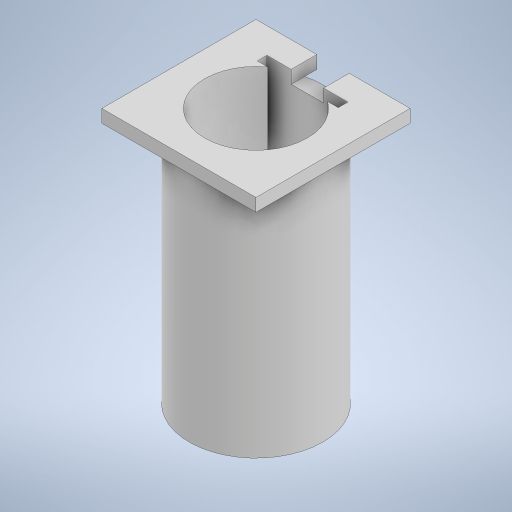
# Autodesk Inventor part: WaterBucket2
Saved by Autodesk Inventor 2023 (Build 270158000, 158)
## iProperties
Created: 2023-11-16
Part Number: WaterBucket2
Material: Generic
Document SubType Name: Modeling
Designer: Gage
Density: 1 g/cm^3
Appearance: Default
Author: Gage
Autodesk Inventor part; units mm, degrees
ref_plane "YZ Plane" through (0, 0, 0) normal (1, 0, 0) x (0, 1, 0)
ref_plane "XZ Plane" through (0, 0, 0) normal (0, 1, 0) x (-1, 0, 0)
ref_plane "XY Plane" through (0, 0, 0) normal (0, 0, 1) x (1, 0, 0)
sketch "Sketch1" plane through (0, 0, 0) normal (0, 1, 0) x (-1, 0, 0)
  circle A0 centre (0, 0) radius 16.51
  dimension "d0" = 33.02
  constraints: 1 centre point, 1 coincident
  measures "d0" diameter of A0
extrude "Extrusion1" add sketch "Sketch1" along normal blind 58.42
sketch "Sketch3" plane through (0, 58.42, 0) normal (0, 1, 0) x (1, 0, 0)
  line L0 (-19.05, 19.05) -> (19.05, 19.05)
  line L1 (19.05, 19.05) -> (19.05, -19.05)
  line L2 (19.05, -19.05) -> (-19.05, -19.05)
  line L3 (-19.05, -19.05) -> (-19.05, 19.05)
  point P0 (0, 0)
  point P1 (19.05, 0)
  point P2 (0, 19.05)
  dimension "d8" = 38.1
  dimension "d9" = 38.1
  constraints: 8 end point, 2 midpoint, 2 parallel, 1 horizontal, 1 horizontal alignment, 1 perpendicular, 1 vertical alignment
  measures "d8" distance of L1.end L2.end
  measures "d9" distance of L0.end L1.end
extrude "Extrusion3" add sketch "Sketch3" along normal blind 3.175
sketch "Sketch4" plane through (0, 61.595, 0) normal (0, 1, 0) x (1, 0, 0)
  circle A0 centre (0, 0) radius 12.7
  line L0 (-10, 12.7) -> (10, 12.7)
  line L1 (10, 12.7) -> (10, 10.3187)
  line L2 (10, 10.3187) -> (-10, 10.3187)
  line L3 (-10, 10.3187) -> (-10, 12.7)
  point P0 (-12.7, 0)
  point P1 (12.7, 0)
  point P2 (0, 12.7)
  point P3 (-7.4036, 10.3187)
  point P4 (7.4036, 10.3187)
  dimension "d12" = 25.4
  dimension "d13" = 20
  dimension "d14" = 2.3813
  constraints: 8 end point, 3 point on circle, 2 parallel, 1 centre point, 1 coincident, 1 horizontal, 1 midpoint, 1 perpendicular, 1 vertical alignment
  measures "d12" diameter of A0
  measures "d13" distance of L1.end L2.end
  measures "d14" distance between parallel lines of L2 L0
extrude "Extrusion4" cut sketch "Sketch4" against normal blind 61.9125
sketch "Sketch5" plane through (19.05, 58.42, -19.05) normal (0, 0, -1) x (-1, 0, 0)
  line L0 (15.05, 0) -> (23.05, 0)
  line L1 (23.05, 0) -> (23.05, 3.175)
  line L2 (23.05, 3.175) -> (15.05, 3.175)
  line L3 (15.05, 3.175) -> (15.05, 0)
  line L4 (0, 0) -> (0, 3.175) projected
  line L5 (0, 3.175) -> (38.1, 3.175) projected
  point P0 (19.05, -58.42)
  point P1 (19.05, 1.5875)
  point P2 (23.05, 1.5875)
  point P3 (19.05, 3.175)
  dimension "d17" = 8
  dimension "d18" = 3.175
  dimension "d20" = 19.05
  dimension "d21" = 0
  constraints: 8 end point, 2 midpoint, 2 parallel, 1 horizontal, 1 horizontal alignment, 1 perpendicular, 1 vertical alignment
  measures "d17" distance of L2.end L1.end
  measures "d18" distance of L1.end L0.end
  measures "d20" distance of L4.end point (19.05, 3.175)
  measures "d21" distance from line of L5 point (19.05, 3.175)
extrude "Extrusion5" cut sketch "Sketch5" against normal blind 12.7
sketch "Sketch6" plane through (0, 0, 0) normal (0, -1, 0) x (1, 0, 0)
  arc A0 (7.4036, -10.3187) -> (-7.4036, -10.3187) centre (0, 0) ccw projected
  circle A1 centre (0, 0) radius 16.51
  constraints: 1 centre point, 1 coincident
extrude "Extrusion6" add sketch "Sketch6" along normal blind 1.5875
body "Solid1"
